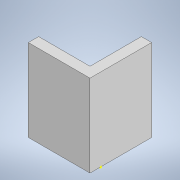
# Autodesk Inventor part: Part11
Saved by Autodesk Inventor 2020 (Build 240168000, 168)
## iProperties
Created: 2019-12-30
Part Number: Part11
Material: Generic
Document SubType Name: Modeling
Designer: tdmp4
Density: 1 g/cm^3
Appearance: Default
Author: tdmp4
Autodesk Inventor part; units mm, degrees
ref_plane "YZ Plane" through (0, 0, 0) normal (1, 0, 0) x (0, 1, 0)
ref_plane "XZ Plane" through (0, 0, 0) normal (0, 1, 0) x (-1, 0, 0)
ref_plane "XY Plane" through (0, 0, 0) normal (0, 0, 1) x (1, 0, 0)
sketch "Sketch1" plane through (0, 0, 0) normal (0, 1, 0) x (-1, 0, 0)
  line L0 (0, 0) -> (19.05, 0)
  line L1 (19.05, 0) -> (19.05, -3.175)
  line L2 (19.05, -3.175) -> (3.175, -3.175)
  line L3 (3.175, -3.175) -> (3.175, -19.05)
  line L4 (3.175, -19.05) -> (0, -19.05)
  line L5 (0, -19.05) -> (0, 0)
  dimension "d0" = 19.05
  dimension "d1" = 3.175
  dimension "d2" = 15.875
  dimension "d3" = 15.875
  constraints: 12 end point, 3 perpendicular, 2 horizontal, 1 vertical
  measures "d0" distance of L0.start L0.end
  measures "d1" distance of L0.end L1.end
  measures "d2" distance of L1.end L2.end
  measures "d3" distance of L2.end L3.end
extrude "Extrusion1" add sketch "Sketch1" along normal blind 25.4
sketch "Sketch2" plane through (-3.175, 0, -3.175) normal (0, 0, -1) x (-1, 0, 0)
  point P0 (-3.175, 0)
body "Solid1"
